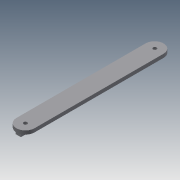
# Autodesk Inventor part: Part4
Saved by Autodesk Inventor 2015 (Build 190159000, 159)
## iProperties
Created: 2014-07-15
Part Number: Part4
Material: Generic
Document SubType Name: Modeling
Designer: shohei
Density: 1 g/cm^3
Appearance: Default
Mass: 197.733 g
Surface Area: 489.325 cm^2
Volume: 197.733 cm^3
Author: shohei
Autodesk Inventor part; units mm, degrees
ref_plane "YZ Plane" through (0, 0, 0) normal (1, 0, 0) x (0, 1, 0)
ref_plane "XZ Plane" through (0, 0, 0) normal (0, 1, 0) x (-1, 0, 0)
ref_plane "XY Plane" through (0, 0, 0) normal (0, 0, 1) x (1, 0, 0)
sketch "Sketch1" plane through (0, 0, 0) normal (0, 0, 1) x (1, 0, 0)
  line L0 (-7.5, 200) -> (7.5, 200)
  line L1 (7.5, 200) -> (7.5, -200)
  line L2 (7.5, -200) -> (-7.5, -200)
  line L3 (-7.5, -200) -> (-7.5, 200)
  line L4 (-35, 0) -> (35, 0) projected
  line L5 (0, -315) -> (0, 315) projected
  line L6 (-25, 200) -> (-25, -200)
  line L7 (25, 200) -> (25, -200)
  arc A0 (25, 200) -> (-25, 200) centre (0, 200) ccw
  arc A1 (-25, -200) -> (25, -200) centre (0, -200) ccw
  point P0 (0, 0)
  dimension "d4" = 7.5
  dimension "d5" = 7.5
  dimension "d6" = 200
  dimension "d7" = 200
  constraints: 12 end point, 4 point on circle, 3 parallel, 2 centre point, 2 midpoint, 2 point on line, 1 horizontal, 1 perpendicular, 1 tangent
  measures "d4" distance between parallel lines of L1 L5
  measures "d5" distance between parallel lines of L3 L5
  measures "d6" distance between parallel lines of L0 L4
  measures "d7" distance between parallel lines of L2 L4
extrude "Extrusion1" add sketch "Sketch1" along normal blind 20 contours L0 L5 L4 L3 | L0 L1 L4 L5 | L4 L5 L2 L3 | L4 L1 L2 L5
sketch "Sketch2" plane through (0, 0, 20) normal (0, 0, 1) x (1, 0, 0)
  circle A0 centre (0, 180) radius 5
  circle A1 centre (0, -180) radius 5
  line L0 (-10.5, 0) -> (10.5, 0) projected
  line L1 (0, -280) -> (0, 280) projected
  point P0 (0, 0)
  dimension "d8" = 10
  dimension "d9" = 180
  dimension "d10" = 180
  dimension "d11" = 10
  constraints: 2 centre point
  measures "d8" diameter of A0
  measures "d9" distance from line of L0 A0.centre
  measures "d10" distance from line of A1.centre L0
  measures "d11" diameter of A1
extrude "Extrusion2" cut sketch "Sketch2" against normal blind 10
sketch "Sketch3" plane through (0, 0, 20) normal (0, 0, 1) x (1, 0, 0)
  circle A0 centre (0, -180) radius 5 projected
  circle A1 centre (0, -180) radius 25
  circle A2 centre (0, 179.3378) radius 25
  line L0 (-25, 179.3378) -> (-25, -180)
  line L1 (25, 179.3378) -> (25, -180)
  point P0 (0, 0)
  dimension "d14" = 50
  dimension "d15" = 50
  constraints: 4 end point, 4 point on circle, 2 centre point, 1 coincident, 1 tangent, 1 vertical
  measures "d14" diameter of A1
  measures "d15" diameter of A2
extrude "Extrusion3" add sketch "Sketch3" against normal blind 20
mirror "Mirror1" about plane through (0, 0, 0) normal (0, 1, 0) of "Extrusion2"
body "Solid1"
